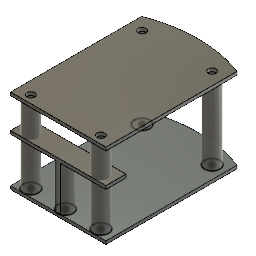
Body (Autodesk Fusion 360 design; units mm, degrees)
Autodesk Fusion 360 part; units mm, degrees
ref_plane "Arbeitsebene1" through (0, -17.5, 0) normal (0, 1, 0) x (0, 0, 1)
sketch "Skizze1" plane through (0, -17.5, 0) normal (0, 1, 0) x (1, 0, 0)
  line L0 (-21.5, 31.5) -> (21.5, 31.5) construction
  line L1 (21.5, 31.5) -> (21.5, -31.5)
  line L2 (21.5, -31.5) -> (-21.5, -31.5)
  line L3 (-21.5, -31.5) -> (-21.5, 31.5)
  arc A0 (21.5, 27.5) -> (-21.5, 27.5) centre (0, -28.2812) ccw
  circle A1 centre (-15.75, -28) radius 1.75
  circle A2 centre (15.75, -28) radius 1.75
  circle A3 centre (15.75, 22) radius 1.75
  circle A4 centre (-15.75, 22) radius 1.75
  dimension "d2" = 43
  dimension "d3" = 21.5
  dimension "d4" = 63
  dimension "d5" = 31.5
  dimension "d6" = 59
  dimension "d9" = 3.5
  dimension "d10" = 3.5
  dimension "d11" = 31.5
  dimension "d12" = 15.75
  dimension "d13" = 50
  constraint horizontal L0
  constraint vertical L1
  constraint horizontal L2
  constraint vertical L3
  constraint tangent L0 A0
  constraint coincident L1 A0.start
  constraint coincident L3 A0.end
  constraint horizontal A0.end A0.start
  constraint equal A1 A4
  constraint equal A1 A2
  constraint equal A1 A3
  constraint vertical A1.centre A4.centre
  constraint vertical A2.centre A3.centre
  constraint horizontal A1.centre A2.centre
  constraint horizontal A3.centre A4.centre
  measures "d2" distance of L1 L3
  measures "d3" distance of origin L1
  measures "d4" distance of L0.end L1.end
  measures "d5" distance of origin L2
  measures "d6" distance of L2 A0.end
  measures "d9" diameter of A1
  measures "d10" distance of L2 A1.centre
  measures "d11" distance of A1.centre A2.centre
  measures "d12" horizontal distance of origin A2.centre
  measures "d13" distance of A2.centre A3.centre
ref_plane "Arbeitsebene2" through (0, 17.5, 0) normal (0, 1, 0) x (0, 0, 1)
sketch "Skizze2" plane through (0, 17.5, 0) normal (0, 1, 0) x (1, 0, 0)
  circle A0 centre (15.75, -28) radius 1.75
  circle A1 centre (15.75, 22) radius 1.75
  circle A2 centre (-15.75, 22) radius 1.75
  circle A3 centre (-15.75, -28) radius 1.75
  line L0 (21.5, -31.5) -> (21.5, 27.5)
  arc A4 (21.5, 27.5) -> (-21.5, 27.5) centre (0, -28.2812) ccw
  line L1 (-21.5, 27.5) -> (-21.5, -31.5)
  line L2 (-21.5, -31.5) -> (21.5, -31.5)
extrude "Extrusion3" add sketch "Skizze2" along normal blind 1.5 makes body 1
extrude "Extrusion4" add sketch "Skizze1" against normal blind 1.5 separate body makes body 2
ref_plane "Arbeitsebene3" through (0, 2.5, -2.1434) normal (0, 1, 0) x (1, 0, 0)
sketch "Skizze3" plane through (0, 2.5, -2.1434) normal (0, 1, 0) x (1, 0, 0)
  line L0 (-21.5, -24.6434) -> (21.5, -24.6434)
  line L1 (21.5, -24.6434) -> (21.5, -33.6434)
  line L2 (21.5, -33.6434) -> (-21.5, -33.6434)
  line L3 (-21.5, -33.6434) -> (-21.5, -24.6434)
  line L4 (-21.5, 25.3566) -> (-21.5, -33.6434)
  line L5 (21.5, -33.6434) -> (21.5, 25.3566)
  line L6 (-21.5, -33.6434) -> (21.5, -33.6434)
  circle A0 centre (-15.75, -30.1434) radius 1.75
  circle A1 centre (15.75, -30.1434) radius 1.75
  dimension "d22" = 9
  constraint horizontal L0
  constraint vertical L1
  constraint horizontal L2
  constraint vertical L3
  constraint collinear L3 L4
  constraint collinear L1 L5
  constraint collinear L2 L6
  measures "d22" distance of L0.start L2.end
extrude "Extrusion6" add sketch "Skizze3" along normal blind 1.5 separate body makes body 3
sketch "Skizze4" plane through (0, -17.5, 0) normal (0, 1, 0) x (-1, 0, 0)
  circle A0 centre (15.75, 28) radius 1.75
  circle A1 centre (-15.75, 28) radius 1.75
  circle A2 centre (15.75, -22) radius 1.75
  circle A3 centre (-15.75, -22) radius 1.75
  line L0 (-21.5, 31.5) -> (-21.5, -27.5)
  arc A4 (-21.5, -27.5) -> (21.5, -27.5) centre (0, 28.2812) ccw
  line L1 (21.5, -27.5) -> (21.5, 31.5)
  line L2 (21.5, 31.5) -> (-21.5, 31.5)
  circle A5 centre (15.75, -22) radius 3.4
  circle A6 centre (-15.75, -22) radius 3.4
  circle A7 centre (15.75, 28) radius 3.4
  circle A8 centre (-15.75, 28) radius 3.4
  circle A9 centre (0, 28.2812) radius 3.4
  dimension "d27" = 6.8
  constraint concentric A2 A5
  constraint concentric A3 A6
  constraint concentric A0 A7
  constraint concentric A1 A8
  constraint concentric A4 A9
  constraint equal A5 A6
  constraint equal A6 A8
  constraint equal A5 A7
  constraint equal A5 A9
  measures "d27" diameter of A5
extrude "Extrusion7" add sketch "Skizze4" along normal blind 35 separate body contours A5 | A6 | A7 | A8 makes body 4 at (-19.1331, 5.8333, 27.6615) makes body 5 at (-19.1331, 5.8333, -22.3385) makes body 6 at (12.3669, 5.8333, 27.6615) makes body 7 at (12.3669, 5.8333, -22.3385)
extrude "Extrusion8" add sketch "Skizze4" along normal blind 20 contours L2 A9 picked at (-0.1387, 27.0692) bodies 2 4 6 3
equation "d1 = ( -35 / 2 ) * 1 mm"
equation "d3 = d2 / 2"
equation "d5 = d4 / 2"
equation "d12 = d11 / 2"
equation "d16 = ( 35 / 2 ) * 1 mm"
